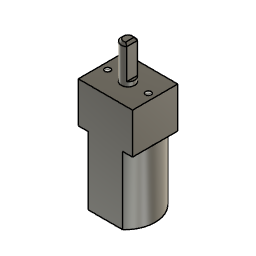
Gripper-3dita v31 (Autodesk Fusion 360 archive; units mm, degrees)
design "motore N20 A2.60RPM"
Autodesk Fusion 360 part; units mm, degrees
sketch "Schizzo1" plane through (0, 0, 0) normal (0, 0, 1) x (1, 0, 0)
  line L0 (-14.6061, 11.2687) -> (-2.6061, 11.2687) construction
  line L1 (-2.6061, 11.2687) -> (-2.6061, 1.2687)
  line L2 (-2.6061, 1.2687) -> (-14.6061, 1.2687) construction
  line L3 (-14.6061, 1.2687) -> (-14.6061, 11.2687)
  line L4 (-12.4061, 11.2687) -> (-4.8061, 11.2687)
  line L5 (-12.4061, 1.2687) -> (-4.8061, 1.2687)
  arc A0 (-12.4061, 11.2687) -> (-12.4061, 1.2687) centre (-7.8242, 6.2687) ccw
  arc A1 (-4.8061, 1.2687) -> (-4.8061, 11.2687) centre (-9.3879, 6.2687) ccw
  line L6 (-14.6061, 11.2687) -> (-2.6061, 1.2687)
  line L7 (-2.6061, 11.2687) -> (-14.6061, 1.2687)
  line L8 (-22.6061, 6.2687) -> (5.3939, 6.2687)
  dimension "d1" = 10
  dimension "d2" = 12
  dimension "d5" = 7.6
  dimension "d6" = 7.6
  constraint horizontal L0
  constraint vertical L1
  constraint horizontal L2
  constraint vertical L3
  constraint coincident L0 L4.start
  constraint parallel L0 L4
  constraint coincident L2 L5.start
  constraint parallel L2 L5
  constraint equal A0 A1
  constraint tangent L3 A0
  constraint tangent L1 A1
  constraint horizontal L8
  constraint midpoint L7 L8
  constraint coincident A1.centre L8
  measures "d1" distance of L0.start L2.end
  measures "d2" distance of L0.start L0.end
  measures "d5" distance of L4.start L4.end
  measures "d6" distance of L5.start L5.end
extrude "Estrusione1" add sketch "Schizzo1" along normal blind 15 contours A1 L7 L8 | A1 L6 L8 | L4 A0 A1 L6 L7 | L5 A0 A1 L6 L7 | A0 L6 L8 | A0 L7 L8
sketch "Schizzo2" plane through (0, 0, 15) normal (0, 0, 1) x (-1, 0, 0)
  arc A0 (12.4061, -11.2687) -> (12.4061, -1.2687) centre (7.8242, -6.2687) ccw
  line L0 (12.4061, -1.2687) -> (4.8061, -1.2687)
  arc A1 (4.8061, -1.2687) -> (4.8061, -11.2687) centre (9.3879, -6.2687) ccw
  line L1 (4.8061, -11.2687) -> (12.4061, -11.2687)
  line L2 (14.6061, -11.2687) -> (2.6061, -11.2687)
  line L3 (2.6061, -11.2687) -> (2.6061, -1.2687)
  line L4 (2.6061, -1.2687) -> (14.6061, -1.2687)
  line L5 (14.6061, -1.2687) -> (14.6061, -11.2687)
  constraint horizontal L2
  constraint vertical L3
  constraint horizontal L4
  constraint vertical L5
  constraint collinear L0 L4
  constraint collinear L1 L2
  constraint tangent A1 L3
  constraint tangent A0 L5
extrude "Estrusione2" add sketch "Schizzo2" along normal blind 9
sketch "Schizzo3" plane through (0, 0, 24) normal (0, 0, 1) x (-1, 0, 0)
  line L0 (14.6061, -1.2687) -> (2.6061, -1.2687)
  line L1 (2.6061, -1.2687) -> (2.6061, -11.2687)
  line L2 (2.6061, -11.2687) -> (14.6061, -11.2687)
  line L3 (14.6061, -11.2687) -> (14.6061, -1.2687)
  line L4 (8.6061, -1.2687) -> (8.6061, -11.2687)
  circle A0 centre (8.6061, -6.2687) radius 1.5
  dimension "d9" = 3
  constraint midpoint L0 L4.start
  constraint midpoint L2 L4.end
  constraint midpoint L4 A0.centre
  measures "d9" diameter of A0
extrude "Estrusione3" add sketch "Schizzo3" along normal blind 1 contours L4 A0 | L4 A0
sketch "Schizzo4" plane through (0, 0, 25) normal (0, 0, 1) x (-1, 0, 0)
  circle A0 centre (8.6061, -6.2687) radius 1.5
  line L0 (7.7061, -7.4687) -> (7.7061, -3.5)
  line L1 (7.7061, -3.5) -> (10.1061, -3.5)
  line L2 (10.1061, -3.5) -> (10.1061, -6.2687)
  arc A1 (7.7061, -7.4687) -> (7.7061, -5.0687) centre (8.6061, -6.2687) ccw
  dimension "d12" = 3
  dimension "d13" = 2.4
  constraint concentric A0 A1
  constraint vertical L0
  constraint horizontal L1
  constraint vertical L2
  constraint tangent L2 A1
  constraint coincident A0 L2.end
  constraint coincident A0 L0.start
  constraint coincident L0 A1.end
  measures "d12" diameter of A1
  measures "d13" distance of L0.end L1.end
extrude "Estrusione4" add sketch "Schizzo4" along normal blind 7.2 contours A0 L0 A1
chamfer "Smusso1" distance 0.5 angle 45 1 faces at (-8.4844, 6.1233, 32.2)
sketch "Schizzo5" plane through (0, 0, 0) normal (0, 0, -1) x (1, 0, 0)
  arc A0 (-12.4061, -1.2687) -> (-12.4061, -11.2687) centre (-7.8242, -6.2687) ccw
  line L0 (-12.4061, -11.2687) -> (-4.8061, -11.2687)
  arc A1 (-4.8061, -11.2687) -> (-4.8061, -1.2687) centre (-9.3879, -6.2687) ccw
  line L1 (-4.8061, -1.2687) -> (-12.4061, -1.2687)
  circle A2 centre (-12.3093, -6.2383) radius 1.5561
  circle A3 centre (-5.3753, -6.1228) radius 1.5561
  constraint equal A2 A3
extrude "Estrusione5" add sketch "Schizzo5" along normal blind 2.039 contours A2 | A3
fillet "Raccordo1" radius 1.5 2 faces at (-12.7379, 6.5305, -2.039) (-4.8514, 6.3478, -2.039)
sketch "Schizzo6" plane through (0, 0, 24) normal (0, 0, 1) x (-1, 0, 0)
  circle A0 centre (8.6061, -6.2687) radius 1.5
  line L0 (14.6061, -1.2687) -> (2.6061, -1.2687)
  line L1 (2.6061, -1.2687) -> (2.6061, -11.2687)
  line L2 (2.6061, -11.2687) -> (14.6061, -11.2687)
  line L3 (14.6061, -11.2687) -> (14.6061, -1.2687)
  line L4 (13.1061, -6.2687) -> (4.1061, -6.2687)
  point P0 (13.1061, -6.2687)
  point P1 (4.1061, -6.2687)
  dimension "d21" = 9
  constraint perpendicular L3 L4
  constraint midpoint A0.centre L4
  constraint coincident P0 L4.start
  constraint coincident P1 L4.end
  measures "d21" distance of P0 P1
hole "Foratura1" at (-13.1061, 6.2687, 24) at (-4.1061, 6.2687, 24) direction (0, 0, -1) diameter 1.271 depth 6 tip angle 118
thread "Filettatura1" "ISO Metric profile 1.6 M1.6x0.35 6H" thread offset 0 thread depth 7.4
